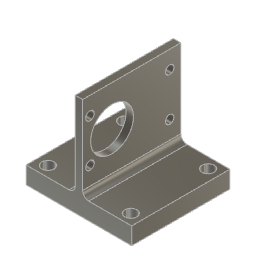
Motor Mount v1 (Autodesk Fusion 360 design; units mm, degrees)
Autodesk Fusion 360 part; units mm, degrees
sketch "Sketch1" plane through (0, 0, 0) normal (1, 0, 0) x (0, 1, 0)
  line L0 (20, 16) -> (-20, 16)
  line L1 (-20, 16) -> (-20, -16)
  line L2 (-20, -16) -> (20, -16)
  line L3 (20, -16) -> (20, 16)
  line L4 (20, 16) -> (-20, -16) construction
  line L5 (-20, 16) -> (20, -16) construction
  line L6 (17, 26.4407) -> (-17, 26.4407)
  line L7 (-17, 26.4407) -> (-17, -26.4407)
  line L8 (-17, -26.4407) -> (17, -26.4407)
  line L9 (17, -26.4407) -> (17, 26.4407)
  line L10 (17, 26.4407) -> (-17, -26.4407) construction
  line L11 (-17, 26.4407) -> (17, -26.4407) construction
  line L12 (55.3865, 8.75) -> (-55.3865, 8.75)
  line L13 (-55.3865, 8.75) -> (-55.3865, -8.75)
  line L14 (-55.3865, -8.75) -> (55.3865, -8.75)
  line L15 (55.3865, -8.75) -> (55.3865, 8.75)
  line L16 (55.3865, 8.75) -> (-55.3865, -8.75) construction
  line L17 (-55.3865, 8.75) -> (55.3865, -8.75) construction
  circle A0 centre (-17, 8.75) radius 1.75
  circle A1 centre (-17, -8.75) radius 1.75
  line L18 (-17, 8.75) -> (-8, 8.75)
  line L19 (-8, 8.75) -> (-8, -9.5577)
  line L20 (-8, -9.5577) -> (-17, -9.5577)
  line L21 (-17, -9.5577) -> (-17, 8.75)
  circle A2 centre (-8, -0.4038) radius 8.7245
  line L22 (17, 8.75) -> (15.5, 8.75)
  line L23 (15.5, 8.75) -> (15.5, -10.3323)
  line L24 (15.5, -10.3323) -> (17, -10.3323)
  line L25 (17, -10.3323) -> (17, 8.75)
  circle A3 centre (15.5, 8.75) radius 1.75
  circle A4 centre (15.5, -8.75) radius 1.75
  dimension "d1" = 40
  dimension "d2" = 32
  dimension "d3" = 34
  dimension "d4" = 17.5
  dimension "d5" = 3.5
  dimension "d7" = 3.5
  dimension "d11" = 9
  dimension "d14" = 1.5
  dimension "d15" = 3.5
  dimension "d16" = 3.5
  constraint horizontal L0
  constraint perpendicular L0 L1
  constraint parallel L0 L2
  constraint parallel L1 L3
  constraint coincident L4 origin
  constraint coincident L5 origin
  constraint horizontal L6
  constraint perpendicular L6 L7
  constraint parallel L6 L8
  constraint parallel L7 L9
  constraint coincident L10 origin
  constraint coincident L11 origin
  constraint horizontal L12
  constraint perpendicular L12 L13
  constraint parallel L12 L14
  constraint parallel L13 L15
  constraint coincident L16 origin
  constraint coincident L17 origin
  constraint coincident L7 A0.centre
  constraint coincident L12 A0.centre
  constraint coincident L7 A1.centre
  constraint coincident L14 A1.centre
  constraint horizontal L18
  constraint vertical L19
  constraint horizontal L20
  constraint vertical L21
  constraint coincident A0.centre L18.start
  constraint midpoint L19 A2.centre
  constraint horizontal L22
  constraint vertical L23
  constraint horizontal L24
  constraint vertical L25
  constraint coincident L22.end L23.start
  constraint coincident L14 A4.centre
  measures "d1" distance of L1.end L2.end
  measures "d2" distance of L0.end L1.end
  measures "d3" distance of L7.end L8.end
  measures "d4" distance of L12.end L13.end
  measures "d5" diameter of A0
  measures "d7" diameter of A1
  measures "d11" distance of A0.centre L18.end
  measures "d14" distance of L22.start L22.end
  measures "d15" diameter of A3
  measures "d16" diameter of A4
extrude "Extrude1" add sketch "Sketch1" along normal blind 3 contours L0 L3 L9 L12 A3 | L0 L7 L9 L12 A0 L18 A3 | L3 L9 L12 L14 L25 A3 A4 | L0 L1 L7 L12 A0 | L9 L12 A3 | L9 L12 L22 A3 | L2 L3 L9 L14 L25 A4 | L9 L12 L25 A3 | L9 L12 L22 L23 L25 A3 | L12 L14 L19 A2 L23 A3 A4 | L12 L23 A3 | L9 L14 L25 A4 | L9 L14 L25 A4 | L9 L23 L25 A3 A4 | L1 L7 L12 L14 A0 A1 L21 | L7 L12 L14 A0 A1 L18 L19 L21 A2 | L2 L7 L9 L14 A1 L19 L20 A2 L24 A4 | L9 L14 L23 L25 A4 | L9 L14 L23 L24 L25 A4 | L9 L24 L25 A4 | L1 L2 L7 L14 A1 | L14 L19 A2 | L14 L19 A2 | L14 L23 A4 | L14 L23 L24 A4 | L14 L19 A2 | L14 L19 A2 | L14 A1 L19 L20 A2
extrude "Extrude2" cut sketch "Sketch1" along normal blind 10 contours L14 L19 A2 | L14 L19 A2 | L14 L19 A2 | L14 L19 A2
extrude "Extrude3" cut sketch "Sketch1" along normal up to surface (3 mm away) contours L9 L12 A3 | L9 L12 L22 A3 | L9 L12 L25 A3 | L9 L12 L22 L23 L25 A3 | L12 L23 A3 | L9 L14 L25 A4 | L9 L14 L25 A4 | L9 L14 L23 L25 A4 | L9 L14 L23 L24 L25 A4 | L14 L23 A4 | L14 L23 L24 A4
extrude "Extrude4" add 1 faces at (1, -6.6667, -16) along direction (0, 0, -1) blind 9.6
sketch "Sketch2" plane through (3, 0, 0) normal (1, 0, 0) x (0, 1, 0)
  circle A0 centre (15.5, 8.75) radius 1.75
  circle A1 centre (15.5, -8.75) radius 1.75
  circle A2 centre (-8, -0.4038) radius 8.7245
  circle A3 centre (-17, -8.75) radius 1.75
  circle A4 centre (-17, 8.75) radius 1.75
  line L0 (20, -25.6) -> (20, 16)
  line L1 (20, 16) -> (-20, 16)
  line L2 (-20, 16) -> (-20, -25.6)
  line L3 (-20, -25.6) -> (20, -25.6)
  line L4 (-20, -25.6) -> (20, -25.6)
  line L5 (20, -25.6) -> (20, -18.6)
  line L6 (20, -18.6) -> (-20, -18.6)
  line L7 (-20, -18.6) -> (-20, -25.6)
  dimension "d21" = 7
  constraint horizontal L4
  constraint vertical L5
  constraint horizontal L6
  constraint vertical L7
  constraint coincident L2.end L3.start
  measures "d21" distance of L2.end L6.end
extrude "Extrude5" add sketch "Sketch2" along normal blind 20 and the other way blind 23 contours L0 L2 L3 L4 L5 L6 L7
sketch "Sketch3" plane through (0, 0, -25.6) normal (0, 0, -1) x (1, 0, 0)
  line L0 (-20, -20) -> (23, -20)
  line L1 (23, -20) -> (23, 20)
  line L2 (23, 20) -> (-20, 20)
  line L3 (-20, 20) -> (-20, -20)
  line L4 (-20, 20) -> (23, -20)
  line L5 (23, 20) -> (-20, -20)
  line L6 (-15.3926, 15.7141) -> (18.3926, 15.7141)
  line L7 (18.3926, 15.7141) -> (18.3926, -15.7141)
  line L8 (18.3926, -15.7141) -> (-15.3926, -15.7141)
  line L9 (-15.3926, -15.7141) -> (-15.3926, 15.7141)
  line L10 (-15.3926, 15.7141) -> (18.3926, -15.7141) construction
  line L11 (18.3926, 15.7141) -> (-15.3926, -15.7141) construction
  circle A0 centre (-15.3926, 15.7141) radius 2.5
  circle A1 centre (18.3926, 15.7141) radius 2.5
  circle A2 centre (18.3926, -15.7141) radius 2.5
  circle A3 centre (-15.3926, -15.7141) radius 2.5
  point P0 (1.5, 0)
  dimension "d26" = 5
  dimension "d27" = 5
  dimension "d28" = 5
  dimension "d29" = 5
  constraint coincident L2.end L3.start
  constraint coincident L0.end L1.start
  constraint coincident L1.end L2.start
  constraint coincident L0.start L3.end
  constraint horizontal L6
  constraint perpendicular L6 L7
  constraint parallel L6 L8
  constraint parallel L7 L9
  constraint coincident L4 L6.start
  constraint coincident L10 P0
  constraint coincident L11 P0
  constraint midpoint L4 P0
  constraint coincident L6.start L9.end
  constraint coincident L6.end L7.start
  constraint coincident L7.end L8.start
  constraint coincident L8.end L9.start
  measures "d26" diameter of A0
  measures "d27" diameter of A1
  measures "d28" diameter of A2
  measures "d29" diameter of A3
extrude "Extrude6" cut sketch "Sketch3" along normal blind -7 and the other way blind 0 contours L5 L9 A3 | L5 L8 A3 | L4 L8 A2 | L4 L7 A2 | L4 L6 A0 | L4 L9 A0 | L5 L9 A3 | L5 L8 A3 | L5 L7 A1 | L5 L6 A1 | L4 L8 A2 | L4 L7 A2 | L4 L6 A0 | L4 L9 A0 | L5 L7 A1 | L5 L6 A1
fillet "Fillet1" radius 2.5 2 edges at (0, 0, -18.6) (3, 0, -18.6)
